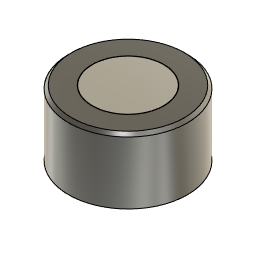
AluminiumPartForTesting (Autodesk Fusion 360 design; units mm, degrees)
Autodesk Fusion 360 part; units mm, degrees
sketch "Skizze1" plane through (0, 0, 0) normal (0, 0, 1) x (1, 0, 0)
sketch "Skizze2" plane through (0, 0, 0) normal (1, 0, 0) x (0, 1, 0)
  line L0 (0, 4) -> (0, 25)
  line L1 (0, 25) -> (12, 25)
  line L2 (12, 25) -> (12, 24)
  line L3 (12, 24) -> (15, 24)
  line L4 (15, 24) -> (15, 23)
  line L5 (15, 23) -> (5.65, 23)
  line L6 (5.65, 23) -> (5.65, 22)
  line L7 (5.65, 22) -> (4, 22)
  line L8 (4, 22) -> (4, 0)
  line L9 (4, 0) -> (2.5, 0)
  line L10 (2.5, 0) -> (2.5, 4)
  line L11 (2.5, 4) -> (0, 4)
  dimension "d2" = 4
  dimension "d4" = 2.5
  dimension "d5" = 4
  dimension "d6" = 15
  dimension "d7" = 3
  dimension "d8" = 1
  dimension "d9" = 1.65
  dimension "d10" = 4
  dimension "d11" = 22
  dimension "d13" = 1
  dimension "d14" = 1
  constraint vertical L0
  constraint perpendicular L0 L1
  constraint perpendicular L1 L2
  constraint perpendicular L2 L3
  constraint perpendicular L3 L4
  constraint perpendicular L4 L5
  constraint perpendicular L5 L6
  constraint perpendicular L0 L7
  constraint perpendicular L5 L8
  constraint perpendicular L8 L9
  constraint perpendicular L9 L10
  constraint perpendicular L0 L11
  measures "d2" distance of L9 L11
  measures "d4" distance of L0 L10
  measures "d5" distance of origin L0.start
  measures "d6" distance of L0 L4
  measures "d7" distance of L2 L4
  measures "d8" distance of L5 L7
  measures "d9" distance of L6.end L7.end
  measures "d10" distance of L0 L8
  measures "d11" distance of L7.end L8.end
  measures "d13" distance of L3.end L4.end
  measures "d14" distance of L1.end L2.end
revolve "Drehen1" add sketch "Skizze2" angle 360 about axis through (0, 0, 1.75) along (0, 0, 1) makes body 1
sketch "Skizze3" plane through (0, 0, 24) normal (0, 0, 1) x (-1, 0, 0)
  circle A0 centre (0, 0) radius 12
  circle A1 centre (0, 0) radius 15
  circle A2 centre (0, 0) radius 12
  circle A3 centre (0, 0) radius 20
  circle A4 centre (0, 0) radius 12.1
  dimension "d15" = 40
  dimension "d16" = 0.1
  constraint concentric A2 A3
  measures "d15" diameter of A3
extrude "Extrusion2" add sketch "Skizze3" along normal blind 1 separate body contours A1 | A3 makes body 2
sketch "Skizze4" plane through (0, 0, 24) normal (0, 0, 1) x (-1, 0, 0)
  circle A0 centre (0, 0) radius 15
  circle A1 centre (0, 0) radius 5.65
  circle A2 centre (0, 0) radius 15.1
  dimension "d21" = 0.1
extrude "Extrusion3" add sketch "Skizze3" against normal blind 1 contours A3 bodies 2
sketch "Skizze5" plane through (0, 0, 23) normal (0, 0, -1) x (1, 0, 0)
  circle A0 centre (0, 0) radius 15
  circle A1 centre (0, 0) radius 20
  circle A2 centre (0, 0) radius 18
  dimension "d24" = -2
extrude "Extrusion4" add sketch "Skizze5" along normal blind 20 contours A1 bodies 2
chamfer "Fase1" distance 1 angle 45 1 edges at (18.6465, 7.2323, 25) on bodies 2
chamfer "Fase2" distance 1 angle 45 1 edges at (-16.7819, -6.5091, 3) on bodies 2
sketch "Skizze6" plane through (0, 0, 22) normal (0, 0, -1) x (1, 0, 0)
  circle A0 centre (0, 0) radius 5.65
  circle A1 centre (0, 0) radius 4
  circle A2 centre (0, 0) radius 4.1
  dimension "d29" = 0.1
extrude "Extrusion5" add sketch "Skizze6" along normal blind 1 separate body contours A0 makes body 3
equation "d5 = d2"
